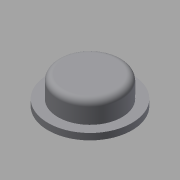
# Autodesk Inventor part: action-button
Saved by Autodesk Inventor 2019 (Build 230136000, 136)
## iProperties
Created: 2019-06-02
Part Number: action-button
Material: Generic
Document SubType Name: Modeling
Designer: jon
Density: 1 g/cm^3
Appearance: Default
Author: jon
Autodesk Inventor part; units mm, degrees
ref_plane "YZ Plane" through (0, 0, 0) normal (1, 0, 0) x (0, 1, 0)
ref_plane "XZ Plane" through (0, 0, 0) normal (0, 1, 0) x (-1, 0, 0)
ref_plane "XY Plane" through (0, 0, 0) normal (0, 0, 1) x (1, 0, 0)
sketch "Sketch1" plane through (0, 0, 0) normal (0, 1, 0) x (-1, 0, 0)
  circle A0 centre (0, 0) radius 5.25
  circle A1 centre (0, 0) radius 4
  dimension "d0" = 10.5
  dimension "d1" = 8
  constraints: 2 centre point, 2 coincident
  measures "d0" diameter of A0
  measures "d1" diameter of A1
extrude "Extrusion1" add sketch "Sketch1" against normal blind 0.8 contours A0 | A1
extrude "Extrusion2" add sketch "Sketch1" along normal blind 2.7 contours A1
fillet "Fillet3" radius 0.75 1 edges at (4, 2.7, 0)
sketch "Sketch2" plane through (0, -0.8, 0) normal (0, -1, 0) x (1, 0, 0)
  arc A0 (0.4286, -2.9692) -> (2.9692, -0.4286) centre (0, 0) ccw
  line L0 (0.4286, -2.9692) -> (0.4286, -0.4286)
  arc A1 (-2.9692, -0.4286) -> (-0.4286, -2.9692) centre (0, 0) ccw
  line L1 (-0.4286, 2.9692) -> (-0.4286, 0.4286)
  arc A2 (-0.4286, 2.9692) -> (-2.9692, 0.4286) centre (0, 0) ccw
  arc A3 (2.9631, 0.4692) -> (0.4286, 2.9692) centre (0, 0) ccw
  line L2 (2.9631, 0.4692) -> (0.4286, 0.4692)
  line L3 (2.9692, -0.4286) -> (0.4286, -0.4286)
  line L4 (0.4286, 0.4692) -> (0.4286, 2.9692)
  line L5 (-0.4286, -0.4286) -> (-0.4286, -2.9692)
  line L6 (-0.4286, -0.4286) -> (-2.9692, -0.4286)
  line L7 (-0.4286, 0.4286) -> (-2.9692, 0.4286)
  circle A4 centre (0, 0) radius 3
  constraints: 16 end point, 9 point on circle, 5 centre point, 4 vertical, 2 horizontal, 1 coincident
extrude "Extrusion3" cut sketch "Sketch2" against normal blind 2 contours L0 L3 A0 | A1 L6 L5 | L2 L4 A3 | A2 L1 L7
body "Solid1"
